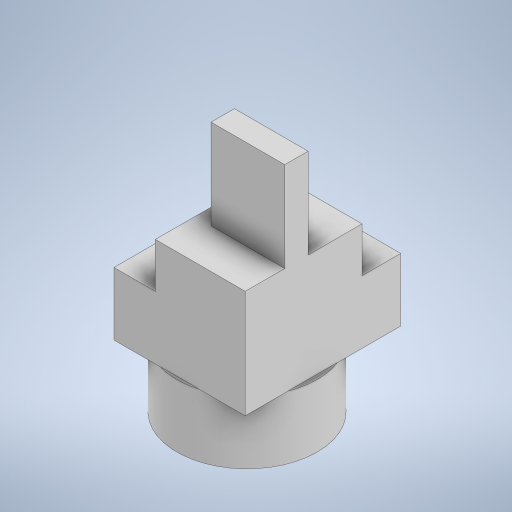
# Autodesk Inventor part: sierr olympic
Saved by Autodesk Inventor 2023 (Build 270158000, 158)
## iProperties
Created: 2022-08-11
Part Number: sierr olympic
Material: Generic
Document SubType Name: Modeling
Designer: Eli
Density: 1 g/cm^3
Appearance: Default
Author: Eli
Autodesk Inventor part; units mm, degrees
ref_plane "YZ Plane" through (0, 0, 0) normal (1, 0, 0) x (0, 1, 0)
ref_plane "XZ Plane" through (0, 0, 0) normal (0, 1, 0) x (-1, 0, 0)
ref_plane "XY Plane" through (0, 0, 0) normal (0, 0, 1) x (1, 0, 0)
sketch "Sketch1" plane through (0, 0, 0) normal (0, 1, 0) x (-1, 0, 0)
  line L0 (0, 0) -> (-37.084, 0)
  line L1 (-37.084, 0) -> (-37.084, -43.942)
  line L2 (-37.084, -43.942) -> (0, -43.942)
  line L3 (0, -43.942) -> (0, 0)
  dimension "d0" = 43.942
  dimension "d1" = 37.084
  constraints: 8 end point, 2 parallel, 1 horizontal, 1 perpendicular
  measures "d0" distance of L2.end L0.start
  measures "d1" distance of L1.end L2.end
extrude "Extrusion1" add sketch "Sketch1" along normal blind 17.78
sketch "Sketch2" plane through (0, 17.78, 0) normal (0, 1, 0) x (1, 0, 0)
  line L0 (0, 0) -> (37.084, 0) projected
  line L1 (37.084, 0) -> (11.684, 0)
  line L2 (11.684, 0) -> (11.684, 33.02)
  line L3 (11.684, 33.02) -> (37.084, 33.02)
  line L4 (37.084, 33.02) -> (37.084, 0)
  dimension "d4" = 33.02
  dimension "d5" = 25.4
  constraints: 8 end point, 2 parallel, 1 horizontal, 1 perpendicular
  measures "d4" distance of L1.end L2.end
  measures "d5" distance of L2.end L3.end
extrude "Extrusion2" add sketch "Sketch2" along normal blind 12.7
sketch "Sketch3" plane through (0, 30.48, 0) normal (0, 1, 0) x (1, 0, 0)
  line L0 (37.084, 0) -> (37.084, 43.942) projected
  line L1 (16.256, 11.176) -> (37.084, 11.176)
  line L2 (37.084, 11.176) -> (37.084, 17.78)
  line L3 (37.084, 17.78) -> (16.256, 17.78)
  line L4 (16.256, 17.78) -> (16.256, 11.176)
  line L5 (11.684, 0) -> (37.084, 0) projected
  point P0 (0, 0)
  dimension "d8" = 17.78
  dimension "d9" = 6.604
  dimension "d10" = 20.828
  constraints: 8 end point, 2 parallel, 1 horizontal, 1 perpendicular, 1 point on line
  measures "d8" distance between parallel lines of L5 L3
  measures "d9" distance of L3.end L1.start
  measures "d10" distance of L2.end L3.end
extrude "Extrusion3" add sketch "Sketch3" along normal blind 25.4
sketch "Sketch4" plane through (0, 0, -43.942) normal (-1, 0, 0) x (0, 0, 1)
  line L0 (7.348, 15.289) -> (38.9211, 15.289) construction
  line L1 (38.9211, 15.289) -> (38.9211, 2.9854) construction
  line L2 (38.9211, 2.9854) -> (7.348, 2.9854) construction
  line L3 (7.348, 2.9854) -> (7.348, 15.289) construction
  point P0 (43.942, 0)
  constraints: 2 other
sketch "Sketch5" plane through (0, 0, 0) normal (0, -1, 0) x (1, 0, 0)
  circle A0 centre (18.542, -19.05) radius 19.812
  line L0 (0, 0) -> (37.084, 0) projected
  line L1 (37.084, -43.942) -> (0, -43.942) construction
  line L2 (18.542, -43.942) -> (18.542, 0) construction
  line L3 (11.684, 0) -> (37.084, 0) construction
  dimension "d13" = 39.624
  dimension "d14" = 19.05
  constraints: 2 end point, 1 centre point, 1 midpoint, 1 perpendicular, 1 point on line
  measures "d13" diameter of A0
  measures "d14" distance from line of L0 A0.centre
extrude "Extrusion4" add sketch "Sketch5" along normal blind 17.78
body "Solid1"
